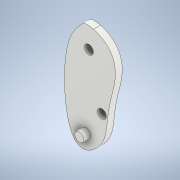
# Autodesk Inventor part: Component35
Saved by Autodesk Inventor 2022 (Build 260153000, 153)
## iProperties
Created: 2022-01-29
Part Number: Component35
Material: Generic
Document SubType Name: Modeling
Designer: Administrator
Density: 1 g/cm^3
Appearance: Default
Title: Component35
Author: Administrator
Autodesk Inventor part; units mm, degrees
ref_plane "YZ Plane" through (0, 0, 0) normal (1, 0, 0) x (0, 1, 0)
ref_plane "XZ Plane" through (0, 0, 0) normal (0, 1, 0) x (-1, 0, 0)
ref_plane "XY Plane" through (0, 0, 0) normal (0, 0, 1) x (1, 0, 0)
sketch "Sketch2" plane through (0, 0, 0) normal (0, 0, 1) x (1, 0, 0)
  circle A0 centre (1.0454, -21.5468) radius 3.25
  circle A1 centre (3.0763, 32.1182) radius 3.25
  circle A2 centre (12.5071, -3.7498) radius 3.25
  spline S0 degree 5 poles (6.4555, 46.5501) (7.8259, 46.1983) (10.7442, 45.2414) (15.3109, 43.005) (19.8831, 38.459) (22.5763, 31.1563) (22.5338, 23.5292) (21.1111, 16.6728) (19.6086, 11.1809) (18.3389, 6.1493) (17.3595, 1.0873) (16.6879, -4.0527) (16.176, -9.1583) (15.5419, -14.078) (14.3136, -18.8471) (11.9682, -23.5862) (8.2436, -28.1103) (3.1985, -31.9372) (-2.1687, -33.4239) (-6.8512, -31.3247) (-10.4942, -25.7174) (-12.9731, -17.2466) (-14.3899, -7.0157) (-14.9009, 3.7736) (-14.5985, 14.1195) (-13.4827, 23.3278) (-11.6061, 30.974) (-9.0323, 36.8714) (-6.1636, 41.1343) (-3.2374, 43.981) (-1.8109, 46.1837) (-0.4485, 47.3092) (2.5216, 47.3522) (5.0851, 46.9019) (6.4555, 46.5501) knots 0 0 0 0 0 0 0.033333 0.066667 0.1 0.133333 0.166667 0.2 0.233333 0.266667 0.3 0.333333 0.366667 0.4 0.433333 0.466667 0.5 0.533333 0.566667 0.6 0.633333 0.666667 0.7 0.733333 0.766667 0.8 0.833333 0.866667 0.9 0.933333 0.966667 1 1 1 1 1 1 weights 1 1 1 1 1 1 1 1 1 1 1 1 1 1 1 1 1 1 1 1 1 1 1 1 1 1 1 1 1 1 1 1 1 1 1
  point P0 (0, 0)
  dimension "d8" = 6.5
  constraints: 3 centre point, 2 equal radius, 1 other
  measures "d8" diameter of A1
extrude "Extrusion1" add sketch "Sketch2" along normal blind 5
sketch "Sketch3" plane through (0, 0, 5) normal (0, 0, 1) x (1, 0, 0)
  circle A0 centre (1.0454, -21.5468) radius 3.25 projected
  circle A1 centre (3.0763, 32.1182) radius 3.25 projected
  circle A2 centre (12.5071, -3.7498) radius 3.25 projected
  point P0 (0, 0)
  point P1 (6.4555, 46.5501)
  constraints: 1 other
extrude "Extrusion2" add sketch "Sketch3" along normal blind 5 contours A0
extrude "Extrusion3" add sketch "Sketch2" along normal blind 5 contours A0
equation "\"d8\" = R"
equation "\"R\" = 6.5"
equation "\"thickness\" = 5"
equation "\"width\" = 6.5"
equation "\"R1\" = 9"
body "Solid1"
